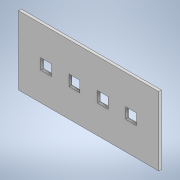
# Autodesk Inventor part: couvercle_contacteur
Saved by Autodesk Inventor 2020.2 (Build 242310000, 310)
## iProperties
Created: 2020-01-15
Part Number: couvercle_contacteur
Material: Générique
Document SubType Name: Modeling
Designer: anton
Density: 1 g/cm^3
Appearance: Par défaut
Author: anton
Autodesk Inventor part; units mm, degrees
ref_plane "YZ Plane" through (0, 0, 0) normal (1, 0, 0) x (0, 1, 0)
ref_plane "XZ Plane" through (0, 0, 0) normal (0, 1, 0) x (-1, 0, 0)
ref_plane "XY Plane" through (0, 0, 0) normal (0, 0, 1) x (1, 0, 0)
sketch "Esquisse1" plane through (0, 0, 0) normal (0, 0, 1) x (1, 0, 0)
  line L0 (-43.1454, 28.8741) -> (60.8546, 28.8741)
  line L1 (60.8546, 28.8741) -> (60.8546, -22.1259)
  line L2 (60.8546, -22.1259) -> (-43.1454, -22.1259)
  line L3 (-43.1454, -22.1259) -> (-43.1454, 28.8741)
  line L4 (-26.6454, 6.8741) -> (-18.6454, 6.8741)
  line L5 (-18.6454, 6.8741) -> (-18.6454, -1.1259)
  line L6 (-18.6454, -1.1259) -> (-26.6454, -1.1259)
  line L7 (-26.6454, -1.1259) -> (-26.6454, 6.8741)
  line L8 (-5.6454, 6.8741) -> (2.3546, 6.8741)
  line L9 (2.3546, 6.8741) -> (2.3546, -1.1259)
  line L10 (2.3546, -1.1259) -> (-5.6454, -1.1259)
  line L11 (-5.6454, -1.1259) -> (-5.6454, 6.8741)
  line L12 (15.3546, 6.8741) -> (23.3546, 6.8741)
  line L13 (23.3546, 6.8741) -> (23.3546, -1.1259)
  line L14 (23.3546, -1.1259) -> (15.3546, -1.1259)
  line L15 (15.3546, -1.1259) -> (15.3546, 6.8741)
  line L16 (36.3546, 6.8741) -> (44.3546, 6.8741)
  line L17 (44.3546, 6.8741) -> (44.3546, -1.1259)
  line L18 (44.3546, -1.1259) -> (36.3546, -1.1259)
  line L19 (36.3546, -1.1259) -> (36.3546, 6.8741)
  point P0 (0, 0)
  dimension "d0" = 51
  dimension "d1" = 104
  dimension "d2" = 8
  dimension "d3" = 8
  dimension "d4" = 8
  dimension "d5" = 8
  dimension "d6" = 8
  dimension "d7" = 8
  dimension "d8" = 8
  dimension "d9" = 8
  dimension "d10" = 16.5
  dimension "d11" = 22
  dimension "d12" = 13
  dimension "d13" = 13
  dimension "d14" = 13
  constraints: 40 end point, 10 parallel, 5 horizontal, 5 perpendicular, 3 point on line
  measures "d0" distance of L2.end L0.start
  measures "d1" distance of L0.start L0.end
  measures "d2" distance of L4.start L4.end
  measures "d3" distance of L6.end L4.start
  measures "d4" distance of L8.start L8.end
  measures "d5" distance of L10.end L8.start
  measures "d6" distance of L12.start L12.end
  measures "d7" distance of L14.end L12.start
  measures "d8" distance of L18.end L16.start
  measures "d9" distance of L16.start L16.end
  measures "d10" distance between parallel lines of L3 L7
  measures "d11" distance between parallel lines of L0 L4
  measures "d12" distance between parallel lines of L11 L5
  measures "d13" distance between parallel lines of L15 L9
  measures "d14" distance between parallel lines of L19 L13
extrude "Extrusion1" add sketch "Esquisse1" along normal blind 2
